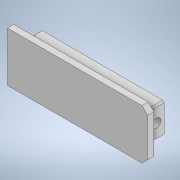
# Autodesk Inventor part: Magazin2_Boden
Saved by Autodesk Inventor 2021 (Build 250183000, 183)
## iProperties
Created: 2024-08-28
Part Number: Magazin2_Boden
Material: Generic
Document SubType Name: Modeling
Designer: Lukas
Density: 1 g/cm^3
Appearance: Default
Author: Lukas
Autodesk Inventor part; units mm, degrees
ref_plane "YZ Plane" through (0, 0, 0) normal (1, 0, 0) x (0, 1, 0)
ref_plane "XZ Plane" through (0, 0, 0) normal (0, 1, 0) x (-1, 0, 0)
ref_plane "XY Plane" through (0, 0, 0) normal (0, 0, 1) x (1, 0, 0)
sketch "Sketch1" plane through (0, 0, 0) normal (0, 0, 1) x (1, 0, 0)
  line L0 (-19.85, 4.85) -> (19.85, 4.85)
  line L1 (19.85, 4.85) -> (19.85, -4.85)
  line L2 (19.85, -4.85) -> (-19.85, -4.85)
  line L3 (-19.85, -4.85) -> (-19.85, 4.85)
  point P0 (0, 0)
  point P1 (0, 4.85)
  point P2 (-19.85, 0)
  dimension "d0" = 39.7
  dimension "d1" = 9.7
  constraints: 8 end point, 2 midpoint, 2 parallel, 1 horizontal, 1 horizontal alignment, 1 perpendicular, 1 vertical alignment
  measures "d0" distance of L0.start L0.end
  measures "d1" distance of L2.end L0.start
extrude "Extrusion1" add sketch "Sketch1" along normal blind 6
sketch "Sketch2" plane through (0, 0, 6) normal (0, 0, 1) x (1, 0, 0)
  line L0 (-22.5, 8) -> (20.7, 8)
  line L1 (20.7, -8) -> (-22.5, -8)
  line L2 (-22.5, -8) -> (-22.5, 8)
  line L3 (20.7, 8) -> (22.5, 6.2)
  line L4 (22.5, 6.2) -> (22.5, -6.2)
  line L5 (22.5, -6.2) -> (20.7, -8)
  line L6 (-19.85, -4.85) -> (19.85, -4.85) projected
  line L7 (19.85, -4.85) -> (19.85, 4.85) projected
  line L8 (19.85, 4.85) -> (-19.85, 4.85) projected
  line L9 (-19.85, 4.85) -> (-19.85, -4.85) projected
  point P0 (0, 0)
  point P1 (-22.5, 0)
  point P2 (22.5, 0)
  dimension "d8" = 16
  dimension "d9" = 45
  dimension "d10" = 22.5
  dimension "d11" = 1.8
  dimension "d12" = 1.8
  constraints: 12 end point, 2 horizontal alignment, 2 midpoint, 2 vertical, 1 horizontal, 1 parallel, 1 perpendicular
  measures "d8" distance of L1.end L0.start
  measures "d9" distance between parallel lines of L4 L2
  measures "d10" distance from line of point (0, 0) L2
  measures "d11" horizontal distance of L0.end L3.end
  measures "d12" horizontal distance of L0.end L3.end
extrude "Extrusion2" add sketch "Sketch2" along normal blind 2 contours L0 L3 L4 L5 L1 L2 | L9 L8 L7 L6
sketch "Sketch3" plane through (-19.85, -4.85, 0) normal (-1, 0, 0) x (0, 0, 1)
  circle A0 centre (2.5, 4.85) radius 1.4
  line L0 (0, 9.7) -> (0, 0) projected
  line L1 (6, 9.7) -> (6, 0) projected
  point P0 (0, 4.85)
  point P1 (0, 4.85)
  dimension "d15" = 3.5
  dimension "d16" = 2.8
  constraints: 1 centre point, 1 horizontal alignment, 1 midpoint
  measures "d15" distance from line of A0.centre L1
  measures "d16" diameter of A0
extrude "Extrusion3" cut sketch "Sketch3" against normal blind 10
mirror "Mirror1" about plane through (0, 0, 0) normal (1, 0, 0) of "Extrusion3"
chamfer "Chamfer1" distance 0.5 angle 45 4 edges at (-19.85, 4.85, 3) (-19.85, -4.85, 3) (19.85, -4.85, 3) (19.85, 4.85, 3)
equation "\"d10\" = 0.5 * d9"
equation "\"d12\" = d11"
body "Solid1"
